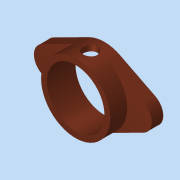
# Autodesk Inventor part: ShaftCollarMagnetMount
Saved by Autodesk Inventor 2017 (Build 210142000, 142)
## iProperties
Created: 2018-04-11
Part Number: ShaftCollarMagnetMount
Material: ABS Plastic
Document SubType Name: Modeling
Designer: Derek Wider
Density: 1.06 g/cm^3
Appearance: Copper - Satin
Author: Derek Wider
Autodesk Inventor part; units mm, degrees
ref_plane "YZ Plane" through (0, 0, 0) normal (1, 0, 0) x (0, 1, 0)
ref_plane "XY Plane" through (0, 0, 0) normal (0, 0, 1) x (1, 0, 0)
sketch "Sketch2" plane through (0, 0, 0) normal (0, 0, 1) x (1, 0, 0)
  circle A0 centre (0, 0) radius 5.05
  circle A1 centre (-7.75, 0) radius 1.55
  circle A2 centre (-7.75, 0) radius 2.5
  circle A3 centre (0, 0) radius 6
  line L0 (-2.7097, 5.3533) -> (-8.879, 2.2305)
  line L1 (-8.879, -2.2305) -> (-2.7097, -5.3533)
  circle A4 centre (7.75, 0) radius 1.55
  circle A5 centre (7.75, 0) radius 2.5
  line L2 (2.7097, 5.3533) -> (8.879, 2.2305)
  line L3 (2.7097, -5.3533) -> (8.879, -2.2305)
  line L4 (0, 0) -> (7.75, 0) construction
  line L5 (0, 0) -> (-7.75, 0) construction
  dimension "d0" = 10.1
  dimension "d1" = 3.1
  dimension "d2" = 5
  dimension "d3" = 12
  dimension "d27" = 7.75
  constraints: 12 end point, 8 point on circle, 8 tangent, 6 centre point, 4 coincident, 2 equal radius, 2 horizontal, 1 collinear
  measures "d0" diameter of A0
  measures "d1" diameter of A1
  measures "d2" diameter of A2
  measures "d3" diameter of A3
  measures "d27" distance of L4.start L4.end
sketch "Sketch5" plane through (0, 0, 0) normal (0, 0, 1) x (1, 0, 0)
  circle A0 centre (0, 0) radius 6 projected
  circle A1 centre (0, 0) radius 5.05 projected
extrude "Extrusion5" add sketch "Sketch5" along normal blind 5
extrude "Extrusion6" add sketch "Sketch2" along normal blind 2 contours A0 | A2 A3 | L0 A3 A2 | A2 A3 L1 | A3 A5 A2 | A2 A3 | L2 A5 A3 | A3 A5 L3 | A5 A3 | A3 A5
sketch "Sketch6" plane through (0, 0, 2) normal (0, 0, 1) x (1, 0, 0)
  circle A0 centre (0, 0) radius 5.05 projected
extrude "Extrusion7" cut sketch "Sketch6" against normal through all
sketch "Sketch7" plane through (0, 0, 2) normal (0, 0, 1) x (1, 0, 0)
  circle A0 centre (-7.75, 0) radius 1.55 projected
  circle A1 centre (7.75, 0) radius 1.55 projected
  point P0 (0, 0)
extrude "Extrusion9" add sketch "Sketch7" against normal blind 0.5
ref_plane "Work Plane3" through (0, 6, 0) normal (0, 1, 0) x (-1, 0, 0)
sketch "Sketch8" plane through (0, 6, 0) normal (0, 1, 0) x (-1, 0, 0)
  line L0 (-5.05, 0) -> (-5.05, 5) projected
  circle A0 centre (0, 2.5) radius 1.25
  point P0 (0, 0)
  point P1 (-5.05, 2.5)
  dimension "d24" = 2.5
  constraints: 1 centre point, 1 horizontal alignment, 1 midpoint
  measures "d24" diameter of A0
extrude "Extrusion10" cut sketch "Sketch8" against normal blind 3
body "Solid2"
